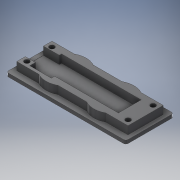
# Autodesk Inventor part: New_Accelite_Controller_Cover_copy_under
Saved by Autodesk Inventor 2018 (Build 220112000, 112)
## iProperties
Created: 2019-03-23
Part Number: New_Accelite_Controller_Cover_copy_under
Material: ABS プラスチック
Document SubType Name: Modeling
Designer: ema
Density: 1.06 g/cm^3
Appearance: 滑らか - 標準の灰色
Author: ema
Autodesk Inventor part; units mm, degrees
ref_plane "YZ Plane" through (0, 0, 0) normal (1, 0, 0) x (0, 1, 0)
ref_plane "XZ Plane" through (0, 0, 0) normal (0, 1, 0) x (-1, 0, 0)
ref_plane "XY Plane" through (0, 0, 0) normal (0, 0, 1) x (1, 0, 0)
sketch "スケッチ1" plane through (0, 0, 0) normal (0, 0, 1) x (1, 0, 0)
  line L0 (-26.25, 10.5) -> (26.25, 10.5)
  line L1 (26.25, 10.5) -> (26.25, -10.5)
  line L2 (26.25, -10.5) -> (-26.25, -10.5)
  line L3 (-26.25, -10.5) -> (-26.25, 10.5)
  point P0 (0, 0)
  dimension "d0" = 52.5
  dimension "d1" = 21
  dimension "d2" = 10.5
  dimension "d3" = 26.25
  constraints: 8 end point, 2 parallel, 1 horizontal, 1 perpendicular
  measures "d0" distance of L0.start L0.end
  measures "d1" distance of L0.end L1.end
  measures "d2" distance from line of L0 point (0, 0)
  measures "d3" distance from line of L1 point (0, 0)
extrude "押し出し1" add sketch "スケッチ1" along normal blind 1.5
sketch "スケッチ6" plane through (0, 0, 1.5) normal (0, 0, 1) x (1, 0, 0)
  line L0 (-24.45, -7.75) -> (-24.45, 7.75)
  line L1 (24.45, 7.75) -> (24.45, -7.75)
  line L2 (24.45, -7.75) -> (14.6971, -7.75)
  arc A0 (14.7186, 7.75) -> (6.2813, 7.75) centre (10.5, -0.0198) ccw
  arc A1 (6.3028, -7.75) -> (14.6971, -7.75) centre (10.5, -0.0198) ccw
  line L3 (14.7186, 7.75) -> (24.45, 7.75)
  line L4 (6.3028, -7.75) -> (-6.2921, -7.75)
  line L5 (-14.7079, -7.75) -> (-24.45, -7.75)
  arc A2 (-6.2921, 7.75) -> (-14.7079, 7.75) centre (-10.5, 0) ccw
  arc A3 (-14.7079, -7.75) -> (-6.2921, -7.75) centre (-10.5, 0) ccw
  line L6 (-24.45, 7.75) -> (-14.7079, 7.75)
  line L7 (-6.2921, 7.75) -> (6.2813, 7.75)
  point P0 (0, 0)
  dimension "d86" = 48.9
  dimension "d87" = 15.5
  dimension "d89" = 24.45
  dimension "d92" = 10.5
  dimension "d93" = 10.5
  dimension "d97" = 15.5
  dimension "d98" = 7.75
  dimension "d99" = 7.75
  dimension "d100" = 7.75
  dimension "d101" = 7.75
  dimension "d102" = 7.75
  dimension "d103" = 57
  dimension "d104" = 57
  dimension "d105" = 57
  dimension "d106" = 57
  constraints: 16 end point, 10 parallel, 8 point on circle, 4 centre point, 3 horizontal, 3 perpendicular
  measures "d86" distance of L1.end L0.start
  measures "d87" distance of L1.start L1.end
  measures "d89" distance from line of point (0, 0) L1
  measures "d92" distance of point (0, 0) A0.centre
  measures "d93" distance of A2.centre point (0, 0)
  measures "d97" distance of L0.start L0.end
  measures "d98" distance from line of L7 point (0, 0)
  measures "d99" distance from line of L4 point (0, 0)
  measures "d100" distance from line of point (0, 0) L2
  measures "d101" distance from line of point (0, 0) L5
  measures "d102" distance from line of A2.centre L6
extrude "押し出し4" add sketch "スケッチ6" along normal blind 3.5
sketch "スケッチ7" plane through (0, 0, 5) normal (0, 0, 1) x (1, 0, 0)
  point P0 (0, 0)
  point P1 (-22.25, 5.5)
  point P2 (-22.25, -5.5)
  point P3 (22.25, 5.5)
  point P4 (22.25, -5.5)
  dimension "d62" = 44.5
  dimension "d63" = 11
  dimension "d64" = 11
  dimension "d65" = 44.5
  dimension "d66" = 22.25
  dimension "d67" = 5.5
  dimension "d68" = 22.25
  dimension "d69" = 5.5
  measures "d62" distance of point (22.25, 5.5) point (-22.25, 5.5)
  measures "d63" distance of point (-22.25, -5.5) point (-22.25, 5.5)
  measures "d64" distance of point (22.25, 5.5) point (22.25, -5.5)
  measures "d65" distance of point (-22.25, -5.5) point (22.25, -5.5)
  measures "d66" horizontal distance of point (0, 0) point (-22.25, 5.5)
  measures "d67" vertical distance of point (-22.25, 5.5) point (0, 0)
  measures "d68" horizontal distance of point (0, 0) point (22.25, -5.5)
  measures "d69" vertical distance of point (0, 0) point (-22.25, -5.5)
hole "穴3" at (-22.25, 5.5, 5) at (-22.25, -5.5, 5) at (22.25, 5.5, 5) at (22.25, -5.5, 5) direction (0, 0, -1) diameter 2.2 end through all
fillet "フィレット3" radius 1 4 edges at (-26.25, -10.5, 0.75) (26.25, -10.5, 0.75) (26.25, 10.5, 0.75) (-26.25, 10.5, 0.75)
sketch "スケッチ8" plane through (0, 0, 5) normal (0, 0, 1) x (1, 0, 0)
  line L0 (-10.5, -5) -> (17.5, -5)
  line L1 (17.5, -5) -> (17.5, 5)
  line L2 (17.5, 5) -> (-17.5, 5)
  line L3 (-24.45, 7.75) -> (-24.45, -7.75) projected
  line L4 (-20, -4) -> (-24.45, -4)
  line L5 (-24.45, -4) -> (-24.45, 4)
  line L6 (-24.45, 4) -> (-17.5, 4)
  line L7 (-25.25, -10.5) -> (25.25, -10.5) projected
  line L8 (25.25, 10.5) -> (-25.25, 10.5) projected
  line L9 (-17.5, 5) -> (-17.5, 4)
  line L10 (-10.5, -5) -> (-10.5, -6.5)
  line L11 (-10.5, -6.5) -> (-17.5, -6.5)
  line L12 (-17.5, -6.5) -> (-20, -6.5)
  line L13 (-20, -6.5) -> (-20, -4)
  point P0 (0, 0)
  dimension "d80" = 35
  dimension "d81" = 10
  dimension "d82" = 5
  dimension "d95" = 6.5
  dimension "d109" = 1.5
  dimension "d111" = 9.5
  constraints: 22 end point, 3 parallel, 2 horizontal, 2 perpendicular, 1 point on line
  measures "d80" distance of L1.end L2.end
  measures "d81" distance of L0.end L1.end
  measures "d82" distance from line of L2 point (0, 0)
  measures "d95" distance between parallel lines of L8 L6
  measures "d109" distance between parallel lines of L0 L11
  measures "d111" distance between parallel lines of L10 L13
extrude "押し出し5" cut sketch "スケッチ8" against normal blind 3.55
equation "\"d2\" = 0.5 * d1"
equation "\"d3\" = 0.5 * d0"
equation "\"d89\" = 0.5 * d86"
equation "\"d93\" = d92"
equation "\"d98\" = 0.5 * d87"
equation "\"d99\" = 0.5 * d97"
equation "\"d100\" = d98"
equation "\"d101\" = d99"
equation "\"d102\" = 0.5 * d97"
equation "\"d64\" = d63"
equation "\"d65\" = d62"
equation "\"d66\" = 0.5 * d62"
equation "\"d67\" = 0.5 * d64"
equation "\"d68\" = d66"
equation "\"d82\" = 0.5 * d81"
equation "\"d95\" = d94"
equation "\"d20\" = 0.5 * d19"
equation "\"d44\" = 0.5 * d43"
equation "\"d55\" = 0.5 * d53"
equation "\"d83\" = 0.5 * d80"
equation "\"d88\" = 0.5 * d87"
equation "\"d94\" = 6.5"
equation "\"d19\" = 14.8"
equation "\"d43\" = 14.8"
equation "\"d53\" = 14.4"
